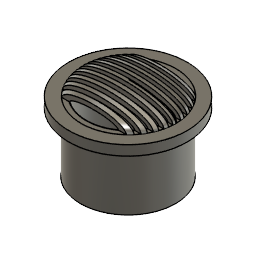
Hot oulet (Autodesk Fusion 360 design; units mm, degrees)
Autodesk Fusion 360 part; units mm, degrees
sketch "Sketch1" plane through (0, 0, 0) normal (0, 0, 1) x (1, 0, 0) in component "sleeve v2 v1"
  circle A0 centre (0, 0) radius 30
  dimension "d1" = 60
  constraint coincident A0.centre origin
  measures "d1" diameter of A0
extrude "Extrude1" add sketch "Sketch1" along normal blind 5 makes body 1 in component "sleeve v2 v1"
sketch "Sketch2" plane through (0, 0, 5) normal (0, 0, 1) x (-1, 0, 0) in component "sleeve v2 v1"
  circle A0 centre (0, 0) radius 30
  circle A1 centre (0, 0) radius 24.1
  dimension "d4" = 48.2
  constraint coincident A0.centre A1.centre
  measures "d4" diameter of A1
extrude "Extrude2" add sketch "Sketch2" along normal blind 25 contours A1 bodies 1 in component "sleeve v2 v1"
sketch "Sketch3" plane through (0, 0, 0) normal (0, 0, -1) x (1, 0, 0) in component "sleeve v2 v1"
  circle A0 centre (0, 0) radius 30
  circle A1 centre (0, 0) radius 24.1
extrude "Extrude3" add sketch "Sketch3" along normal blind 30 contours A1 bodies 1 in component "sleeve v2 v1"
sketch "Sketch4" plane through (0, 0, 30) normal (0, 0, 1) x (-1, 0, 0) in component "sleeve v2 v1"
  circle A0 centre (0, 0) radius 24.1
  circle A1 centre (0, 0) radius 21.1
  dimension "d9" = -3
extrude "Extrude4" cut sketch "Sketch4" against normal blind 60 contours A1 bodies 1 in component "sleeve v2 v1"
extrude "Extrude5" cut 1 faces at (-23.0103, 1.1973, 30) along direction (0, 0, -1) blind 25 on bodies 1 bodies 1 in component "sleeve v2 v1"
sketch "Sketch2 (2)" plane through (0, 0, 0) normal (0, 0, 1) x (1, 0, 0)
  ellipse E0 centre (0, 4.5) end of major axis (21.5, 4.5) minor radius 5 (21.5, 4.5) -> (0, 9.5) ccw
  line L0 (0, 12) -> (0, 9.5)
  line L1 (23.9998, 4.4698) -> (21.5, 4.5)
  ellipse E1 centre (0, 4.5) end of major axis (24, 4.5) minor radius 7.5 (23.9998, 4.4698) -> (0, 12) ccw
  dimension "d18" = 43
  dimension "d54" = 48
  dimension "d55" = 15
  constraint concentric E0 E1
  measures "d18" distance of E0
  measures "d54" distance of E1
revolve "Revolve2" add sketch "Sketch2 (2)" angle 360 about axis through (0, 1.75, 0) along (0, 1, 0) separate body makes body 2
sketch "Sketch3 (2)" plane through (0, 4.7273, 0) normal (0, -1, 0) x (1, 0, 0)
  line L0 (-25, -10.5) -> (27.9885, -10.5)
  line L1 (27.9885, -10.5) -> (27.9885, -8.5)
  line L2 (27.9885, -8.5) -> (-25, -8.5)
  line L3 (-25, -8.5) -> (-25, -10.5)
  line L4 (-25, -6.5) -> (27.9885, -6.5)
  line L5 (-25, -4.5) -> (-25, -6.5)
  line L6 (27.9885, -6.5) -> (27.9885, -4.5)
  line L7 (27.9885, -4.5) -> (-25, -4.5)
  line L8 (27.9885, -0.5) -> (-25, -0.5)
  line L9 (-25, -2.5) -> (27.9885, -2.5)
  line L10 (27.9885, -2.5) -> (27.9885, -0.5)
  line L11 (-25, -0.5) -> (-25, -2.5)
  line L12 (27.9885, 1.5) -> (27.9885, 3.5)
  line L13 (-25, 3.5) -> (-25, 1.5)
  line L14 (-25, 1.5) -> (27.9885, 1.5)
  line L15 (27.9885, 3.5) -> (-25, 3.5)
  line L16 (27.9885, 7.5) -> (-25, 7.5)
  line L17 (-25, 7.5) -> (-25, 5.5)
  line L18 (-25, 5.5) -> (27.9885, 5.5)
  line L19 (27.9885, 5.5) -> (27.9885, 7.5)
  line L20 (27.9885, 9.5) -> (27.9885, 11.5)
  line L21 (-25, 9.5) -> (27.9885, 9.5)
  line L22 (27.9885, 11.5) -> (-25, 11.5)
  line L23 (-25, 15.5) -> (-25, 13.5)
  line L24 (-25, 11.5) -> (-25, 9.5)
  line L25 (-25, 19.5) -> (-25, 17.5)
  line L26 (27.9885, 17.5) -> (27.9885, 19.5)
  line L27 (27.9885, 19.5) -> (-25, 19.5)
  line L28 (-25, 17.5) -> (27.9885, 17.5)
  line L29 (27.9885, 13.5) -> (27.9885, 15.5)
  line L30 (-25, 13.5) -> (27.9885, 13.5)
  line L31 (27.9885, 15.5) -> (-25, 15.5)
  line L32 (27.9885, -12.5) -> (-25, -12.5)
  line L33 (-25, -18.5) -> (27.9885, -18.5)
  line L34 (-25, -14.5) -> (27.9885, -14.5)
  line L35 (-25, -16.5) -> (-25, -18.5)
  line L36 (27.9885, -16.5) -> (-25, -16.5)
  line L37 (-25, -12.5) -> (-25, -14.5)
  line L38 (27.9885, -14.5) -> (27.9885, -12.5)
  line L39 (27.9885, -18.5) -> (27.9885, -16.5)
  circle A0 centre (0, 0.2727) radius 21.1
  circle A1 centre (0, 0.2727) radius 30
  line L40 (27.9885, -22.5) -> (27.9885, -18.5)
  line L41 (-25, -22.5) -> (27.9885, -22.5)
  line L42 (27.9885, -18.5) -> (-25, -18.5)
  line L43 (-25, -18.5) -> (-25, -22.5)
  line L44 (-25, -24.5) -> (27.9885, -24.5)
  line L45 (27.9885, -24.5) -> (27.9885, -22.5)
  line L46 (27.9885, -22.5) -> (-25, -22.5)
  line L47 (-25, -22.5) -> (-25, -24.5)
  line L48 (27.9885, 23.5) -> (-25, 23.5)
  line L49 (-25, 19.5) -> (27.9885, 19.5)
  line L50 (-25, 23.5) -> (-25, 19.5)
  line L51 (27.9885, 19.5) -> (27.9885, 23.5)
  line L52 (27.9885, 23.5) -> (27.9885, 25.5)
  line L53 (-25, 23.5) -> (27.9885, 23.5)
  line L54 (-25, 25.5) -> (-25, 23.5)
  line L55 (27.9885, 25.5) -> (-25, 25.5)
  point P0 (0, 7)
  point P1 (0, 7)
  point P2 (0, 14)
  point P3 (0, 14)
  point P4 (0, 20)
  point P5 (0, 32)
  point P6 (0, 32)
  point P7 (0, -17)
  point P8 (0, -17)
  point P9 (0, -21)
  point P10 (0, -21)
  point P11 (0, -23)
  point P12 (0, -23)
  point P13 (0, 22)
  point P14 (0, 26)
  dimension "d20" = 2
  dimension "d21" = 2
  dimension "d22" = 2
  dimension "d23" = 2
  dimension "d24" = 2
  dimension "d25" = 2.5
  dimension "d26" = 2
  dimension "d27" = 2
  dimension "d28" = 2
  dimension "d29" = 2
  dimension "d30" = 2
  dimension "d31" = 2
  dimension "d32" = 2
  dimension "d36" = 2
  dimension "d37" = 2
  dimension "d40" = 2
  dimension "d44" = 2
  dimension "d45" = 2
  dimension "d50" = 2
  dimension "d51" = 2
  dimension "d56" = 4
  dimension "d57" = 2
  dimension "d58" = 4
  dimension "d59" = 2.5
  dimension "d61" = 2
  dimension "d62" = 2.5
  constraint horizontal L0
  constraint vertical L1
  constraint horizontal L2
  constraint vertical L3
  constraint horizontal L4
  constraint vertical L6
  constraint horizontal L7
  constraint vertical L5
  constraint horizontal L9
  constraint vertical L10
  constraint horizontal L8
  constraint vertical L11
  constraint horizontal L14
  constraint vertical L12
  constraint horizontal L15
  constraint vertical L13
  constraint horizontal L18
  constraint vertical L19
  constraint horizontal L16
  constraint vertical L17
  constraint horizontal L21
  constraint vertical L20
  constraint horizontal L22
  constraint vertical L24
  constraint horizontal L30
  constraint vertical L29
  constraint horizontal L31
  constraint vertical L23
  constraint horizontal L28
  constraint vertical L26
  constraint horizontal L27
  constraint vertical L25
  constraint vertical L39
  constraint vertical L35
  constraint horizontal L34
  constraint vertical L38
  constraint horizontal L32
  constraint vertical L37
  constraint vertical L40
  constraint vertical L43
  constraint vertical L45
  constraint vertical L47
  constraint horizontal L49
  constraint vertical L51
  constraint horizontal L48
  constraint vertical L50
  constraint horizontal L53
  constraint vertical L52
  constraint horizontal L55
  constraint vertical L54
  constraint collinear L27 L49
  measures "d20" distance of L0.start L2.end
  measures "d21" distance of L4.start L5.start
  measures "d22" distance of L9.start L8.end
  measures "d23" distance of L13.end L13.start
  measures "d24" distance of L17.end L16.end
  measures "d25" distance of origin L9
  measures "d26" distance of L7 L9
  measures "d27" distance of L2 L4
  measures "d28" distance of L8 L14
  measures "d29" distance of L15 L18
  measures "d30" distance of L21.start L22.end
  measures "d31" distance of L23.end L23.start
  measures "d32" distance of L25.end L25.start
  measures "d36" distance of L28 L31
  measures "d37" distance of L22 L30
  measures "d40" distance of L16 L21
  measures "d44" distance of L33.start L35.start
  measures "d45" distance of L34.start L32.end
  measures "d50" distance of L34 L36
  measures "d51" distance of L0 L32
  measures "d56" distance of L41.start L33.start
  measures "d57" distance of L44.start L41.start
  measures "d58" distance of L25.start L48.end
  measures "d59" distance of P13 L49
  measures "d61" distance of L48.end L54.start
  measures "d62" distance of P14 L53
extrude "Extrude1'" cut sketch "Sketch3 (2)" against normal blind 15 contours L0 L2 L3 A0 | L0 L2 A0 | L0 L1 L2 A0 | L32 L34 L37 A0 | L32 L34 A0 | L32 L34 A0 A1 | L4 L7 A0 | L4 L5 L7 A0 | L32 L34 L38 A1 | L4 L6 L7 A0 | L33 L36 A0 A1 L42 | L33 L36 A0 L42 | L33 L36 A0 A1 L42 | L8 L9 A0 | L8 L9 L11 A0 | L33 L35 L36 A1 L42 | L33 A0 A1 L41 L42 L46 | L33 A0 L42 | L33 L36 L39 A1 L42 | L20 L22 A1 | L20 L21 L22 A0 A1 | L8 L9 L10 A0 | L27 L28 A0 A1 L49 | L25 L27 L28 A1 L49 | L33 A1 L41 L42 L43 L46 | L33 A1 L40 L41 L42 L46 | L14 L15 A0 | L13 L14 L15 A0 | L27 L28 A0 L49 | L27 A0 A1 L48 L49 L53 | L27 A1 L48 L49 L50 L53 | A1 L41 L44 L46 | A1 L41 L44 L46 L47 | A1 L41 L44 L45 L46 | L21 L22 A0 | L29 L30 L31 A1 | L30 L31 A0 A1 | L12 L14 L15 A0 | L27 L28 A0 A1 L49 | L27 A0 L49 | L23 L30 L31 A0 | L30 L31 A0 | A1 L48 L53 L54 L55 | A1 L48 L53 L55 | L21 L22 L24 A0 | L16 L18 A0 | L16 L18 L19 A0 | L16 L17 L18 A0 | L26 L27 L28 A1 L49 | L27 A1 L48 L49 L51 L53 | A1 L48 L52 L53 L55 bodies 2
component "sleeve v2 v1" placed x (1, 0, 0) y (0, 0, -1) z (0, 1, 0) at (0, -0.2727, 0.2727)
